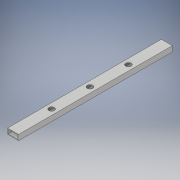
# Autodesk Inventor part: 1x2x28
Saved by Autodesk Inventor 2019 (Build 230136000, 136)
## iProperties
Created: 2018-11-11
Part Number: 1x2x28
Material: Generic
Document SubType Name: Modeling
Designer: maste
Density: 1 g/cm^3
Appearance: Default
Author: maste
Autodesk Inventor part; units mm, degrees
ref_plane "YZ Plane" through (0, 0, 0) normal (1, 0, 0) x (0, 1, 0)
ref_plane "XZ Plane" through (0, 0, 0) normal (0, 1, 0) x (-1, 0, 0)
ref_plane "XY Plane" through (0, 0, 0) normal (0, 0, 1) x (1, 0, 0)
sketch "Sketch1" plane through (0, 0, 0) normal (0, 0, 1) x (1, 0, 0)
  line L0 (0, 0) -> (50.8, 0)
  line L1 (50.8, 0) -> (50.8, 25.4)
  line L2 (50.8, 25.4) -> (0, 25.4)
  line L3 (0, 25.4) -> (0, 0)
  line L4 (3.175, 22.225) -> (47.625, 22.225)
  line L5 (47.625, 22.225) -> (47.625, 3.175)
  line L6 (47.625, 3.175) -> (3.175, 3.175)
  line L7 (3.175, 3.175) -> (3.175, 22.225)
  dimension "d0" = 50.8
  dimension "d1" = 25.4
  dimension "d2" = 3.175
  constraints: 16 end point, 4 parallel, 2 perpendicular, 1 horizontal, 3 other
  measures "d0" distance of L2.end L1.end
  measures "d1" distance of L1.end L0.end
  measures "d2" distance between parallel lines of L2 L4
extrude "Extrusion1" add sketch "Sketch1" along normal blind 711.2
sketch "Sketch2" plane through (0, 25.4, 0) normal (0, 1, 0) x (1, 0, 0)
  line L0 (0, 0) -> (0, -711.2) projected
  line L1 (0, -355.6) -> (50.8, -355.6)
  line L2 (50.8, 0) -> (50.8, -711.2) projected
  line L3 (50.8, -711.2) -> (0, -711.2) projected
  line L4 (0, -355.6) -> (0, -711.2)
  line L5 (0, -533.4) -> (50.8, -533.4)
  line L6 (0, -355.6) -> (0, 0)
  line L7 (0, -177.8) -> (50.8, -177.8)
  circle A0 centre (25.4, -533.4) radius 12.7
  circle A1 centre (25.4, -355.6) radius 12.7
  circle A2 centre (25.4, -177.8) radius 12.7
  dimension "d5" = 25.4
  constraints: 10 end point, 7 midpoint, 3 centre point, 2 perpendicular, 2 point on line, 1 collinear, 1 vertical
  measures "d5" diameter of A0
extrude "Extrusion2" cut sketch "Sketch2" against normal blind 25.4 contours A2 L7 | L7 A2 | A1 L1 | L1 A1 | A0 L5 | L5 A0
body "Solid1"
